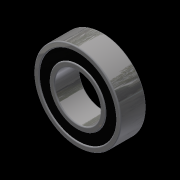
# Autodesk Inventor part: 689-2RS
Saved by Autodesk Inventor 2014 SP1 (Build 180222100, 222)
## iProperties
Created: 2014-05-04
Part Number: 689-2RS
Material: Generic
Document SubType Name: Modeling
Designer: Rauhul Varma
Density: 1 g/cm^3
Appearance: Default
Author: Rauhul Varma
Autodesk Inventor part; units mm, degrees
ref_plane "YZ Plane" through (0, 0, 0) normal (1, 0, 0) x (0, 1, 0)
ref_plane "XZ Plane" through (0, 0, 0) normal (0, 1, 0) x (-1, 0, 0)
ref_plane "XY Plane" through (0, 0, 0) normal (0, 0, 1) x (1, 0, 0)
sketch "Sketch1" plane through (0, 0, 0) normal (0, 0, 1) x (1, 0, 0)
  circle A0 centre (0, 0) radius 4.5
  circle A1 centre (0, 0) radius 8.5
  circle A2 centre (0, 0) radius 5.5
  circle A3 centre (0, 0) radius 7.5
  dimension "d0" = 9
  dimension "d1" = 17
  dimension "d2" = 11
  dimension "d3" = 15
  constraints: 4 centre point, 4 coincident
  measures "d0" diameter of A0
  measures "d1" diameter of A1
  measures "d2" diameter of A2
  measures "d3" diameter of A3
extrude "Extrusion1" add sketch "Sketch1" along normal mid plane 5
extrude "Extrusion2" add sketch "Sketch1" along normal mid plane 4.6031 contours A3
fillet "Fillet1" radius 0.2 8 edges at (-8.5, 0, 2.5) (-7.5, 0, 2.5) (-5.5, 0, 2.5) (-4.5, 0, 2.5) (-8.5, 0, -2.5) (-7.5, 0, -2.5) (-5.5, 0, -2.5) (-4.5, 0, -2.5)
body "Solid1"
